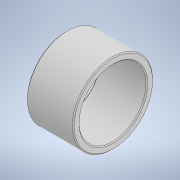
# Autodesk Inventor part: Скольжение
Saved by Autodesk Inventor 2021 (Build 250183000, 183)
## iProperties
Created: 2023-04-27
Part Number: Скольжение
Material: Типовые
Document SubType Name: Modeling
Designer: gdevc
Density: 1 g/cm^3
Appearance: По умолчанию
Author: gdevc
Autodesk Inventor part; units mm, degrees
ref_plane "YZ Plane" through (0, 0, 0) normal (1, 0, 0) x (0, 1, 0)
ref_plane "XZ Plane" through (0, 0, 0) normal (0, 1, 0) x (-1, 0, 0)
ref_plane "XY Plane" through (0, 0, 0) normal (0, 0, 1) x (1, 0, 0)
sketch "Эскиз1" plane through (0, 0, 0) normal (0, 0, 1) x (1, 0, 0)
  line L0 (0, 0) -> (37.7119, 0)
  line L1 (0, 25) -> (35, 25)
  line L2 (0, 30) -> (35, 30)
  line L3 (0, 30) -> (0, 25)
  line L4 (35, 30) -> (35, 25)
  dimension "d0" = 50
  dimension "d1" = 35
  dimension "d3" = 60
  constraints: 10 end point, 2 horizontal, 2 vertical, 1 parallel, 1 point on line
  measures "d0" diameter of L1 L0
  measures "d1" distance of L1.end L1.start
  measures "d3" diameter of L2 L0
revolve "Вращение1" add sketch "Эскиз1" angle 360 about axis through (0, 0, 0) along (1, 0, 0)
chamfer "Фаска1" distance 0.7 angle 45 4 edges at (35, -30, 0) (35, -25, 0) (0, -25, 0) (0, -30, 0)
